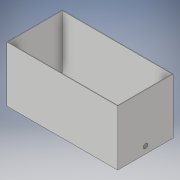
# Autodesk Inventor part: Burner
Saved by Autodesk Inventor 2017 (Build 210142000, 142)
## iProperties
Created: 2018-10-22
Part Number: Burner
Material: Generic
Document SubType Name: Modeling
Designer: mcgratta
Density: 1 g/cm^3
Appearance: Default
Author: mcgratta
Autodesk Inventor part; units mm, degrees
ref_plane "YZ Plane" through (0, 0, 0) normal (1, 0, 0) x (0, 1, 0)
ref_plane "XZ Plane" through (0, 0, 0) normal (0, 1, 0) x (-1, 0, 0)
ref_plane "XY Plane" through (0, 0, 0) normal (0, 0, 1) x (1, 0, 0)
sketch "Sketch1" plane through (0, 0, 0) normal (0, 1, 0) x (-1, 0, 0)
  line L0 (0, 0) -> (609.6, 0)
  line L1 (609.6, 0) -> (609.6, -304.8)
  line L2 (609.6, -304.8) -> (0, -304.8)
  line L3 (0, -304.8) -> (0, 0)
  dimension "d0" = 304.8
  dimension "d1" = 609.6
  constraints: 8 end point, 2 parallel, 1 horizontal, 1 perpendicular
  measures "d0" distance between parallel lines of L2 L0
  measures "d1" distance between parallel lines of L3 L1
extrude "Extrusion1" add sketch "Sketch1" along normal blind 3.175
sketch "Sketch2" plane through (0, 3.175, 0) normal (0, 1, 0) x (1, 0, 0)
  line L0 (-609.6, 0) -> (0, 0) projected
  line L1 (0, 0) -> (0, 304.8) projected
  line L2 (-609.6, 0) -> (0, 0)
  line L3 (0, 0) -> (0, 304.8)
  line L4 (0, 304.8) -> (-609.6, 304.8)
  line L5 (-609.6, 304.8) -> (-609.6, 0)
  line L6 (-606.425, 3.175) -> (-3.175, 3.175)
  line L7 (-3.175, 3.175) -> (-3.175, 301.625)
  line L8 (-3.175, 301.625) -> (-606.425, 301.625)
  line L9 (-606.425, 301.625) -> (-606.425, 3.175)
  dimension "d4" = 3.175
  dimension "d5" = 3.175
  dimension "d6" = 3.175
  dimension "d7" = 3.175
  constraints: 16 end point, 4 parallel, 2 horizontal, 2 perpendicular
  measures "d4" distance between parallel lines of L1 L7
  measures "d5" distance between parallel lines of L0 L6
  measures "d6" distance between parallel lines of L8 L4
  measures "d7" distance between parallel lines of L9 L5
extrude "Extrusion2" add sketch "Sketch2" along normal blind 301.625
sketch "Sketch5" plane through (0, 0, 0) normal (1, 0, 0) x (0, 0, -1)
  circle A0 centre (152.4, 38.1) radius 12.7
  line L0 (304.8, 0) -> (0, 0) projected
  line L1 (304.8, 0) -> (304.8, 304.8) projected
  dimension "d18" = 25.4
  dimension "d19" = 38.1
  dimension "d20" = 152.4
  constraints: 1 centre point
  measures "d18" diameter of A0
  measures "d19" distance from line of L0 A0.centre
  measures "d20" distance from line of L1 A0.centre
extrude "Extrusion5" cut sketch "Sketch5" against normal blind 25.4
body "Solid1"
